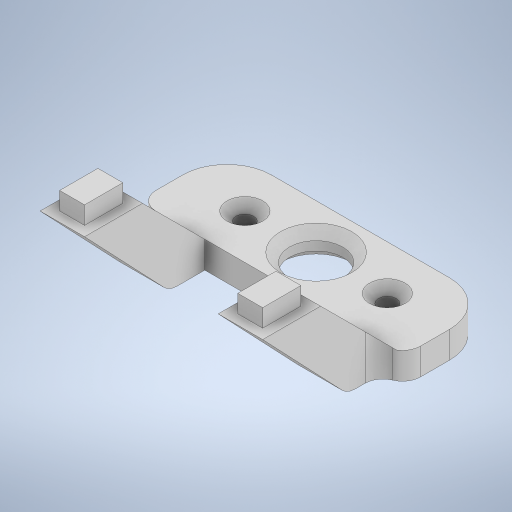
# Autodesk Inventor part: ServoUltrasonicMount
Saved by Autodesk Inventor 2024.2 (Build 282272000, 272)
## iProperties
Created: 2024-04-03
Part Number: ServoUltrasonicMount
Material: Generic
Document SubType Name: Modeling
Designer: ringl
Density: 1 g/cm^3
Appearance: Default
Author: ringl
Autodesk Inventor part; units mm, degrees
ref_plane "XZ Plane" through (0, 0, 0) normal (0, 1, 0) x (-1, 0, 0)
ref_plane "XY Plane" through (0, 0, 0) normal (0, 0, 1) x (1, 0, 0)
sketch "Sketch1" plane through (0, 0, 0) normal (0, 1, 0) x (-1, 0, 0)
  line L0 (0, 0) -> (30, 0)
  line L1 (30, 0) -> (30, -10)
  line L2 (30, -10) -> (0, -10)
  line L3 (0, -10) -> (0, 0)
  dimension "d0" = 30
  dimension "d1" = 10
  constraints: 8 end point, 2 parallel, 1 horizontal, 1 perpendicular
  measures "d0" distance of L1.end L2.end
  measures "d1" distance of L0.end L1.end
extrude "Extrusion1" add sketch "Sketch1" along normal blind 3
ref_plane "Work Plane2" through (-2.5, 0, 0) normal (1, 0, 0) x (0, 1, 0)
sketch "Sketch3" plane through (-2.5, 0, 0) normal (1, 0, 0) x (0, 1, 0)
  line L0 (3, -10) -> (3, 0) projected
  line L1 (3, 0) -> (10, 7)
  line L2 (10, 7) -> (10, 13.5)
  line L3 (10, 13.5) -> (0, 4)
  line L4 (0, 4) -> (0, 0)
  line L5 (0, 0) -> (3, 0) projected
  line L6 (3, 0) -> (0, 0)
  dimension "d13" = 4
  dimension "d14" = 6.5
  dimension "d15" = 45
  dimension "d16" = 10
  constraints: 10 end point, 2 parallel, 1 horizontal
  measures "d13" distance of L3.end L4.end
  measures "d14" distance of L1.end L2.end
  measures "d15" angle of L4 L1
  measures "d16" distance between parallel lines of L4 L2
extrude "Extrusion3" add sketch "Sketch3" against normal blind 5
ref_plane "Work Plane3" through (-15, 0, 0) normal (1, 0, 0) x (0, 1, 0)
fillet "Fillet2" radius 2 1 edges at (-5, 0, 4)
fillet "Fillet3" radius 2 4 edges at (-30, 1.5, 0) (-7.5, 1.5, 0) (-2.5, 1.5, 0) (0, 1.5, 0)
fillet "Fillet4" radius 5 2 edges at (-30, 1.5, -10) (0, 1.5, -10)
sketch "Sketch5" plane through (-2.5, 10, 13.5) normal (0, 1, 0) x (1, 0, 0)
  line L0 (-1.1, 5.4) -> (-3.9, 5.4)
  line L1 (-3.9, 5.4) -> (-3.9, 1.1)
  line L2 (-3.9, 1.1) -> (-1.1, 1.1)
  line L3 (-1.1, 1.1) -> (-1.1, 5.4)
  line L4 (-5, 0) -> (-5, 6.5) projected
  line L5 (0, 6.5) -> (-5, 6.5) projected
  point P0 (2.5, 13.5)
  dimension "d26" = 2.8
  dimension "d27" = 4.3
  dimension "d28" = 1.1
  dimension "d29" = 1.1
  constraints: 8 end point, 2 parallel, 1 horizontal, 1 perpendicular
  measures "d26" distance of L2.end L1.end
  measures "d27" distance of L1.end L0.end
  measures "d28" distance between parallel lines of L4 L1
  measures "d29" distance between parallel lines of L5 L0
extrude "Extrusion4" add sketch "Sketch5" along normal blind 2
mirror "Mirror2" about plane through (-15, 0, 0) normal (1, 0, 0) of "Extrusion3", "Extrusion4"
sketch "Sketch6" plane through (0, 3, 0) normal (0, 1, 0) x (1, 0, 0)
  circle A0 centre (-15, 5) radius 3
  line L0 (-5, 10) -> (-25, 10) projected
  line L1 (0, 1.7081) -> (0, 5) projected
  point P0 (0, 0)
  dimension "d32" = 6
  dimension "d33" = 5
  dimension "d34" = 15
  constraints: 1 centre point
  measures "d32" diameter of A0
  measures "d33" distance from line of L0 A0.centre
  measures "d34" distance from line of A0.centre L1
extrude "Extrusion5" cut sketch "Sketch6" against normal through all
chamfer "Chamfer1" distance 1 angle 45 1 edges at (-18, 3, -5)
sketch "Sketch7" plane through (0, 3, 0) normal (0, 1, 0) x (1, 0, 0)
  circle A0 centre (-23, 5) radius 1
  circle A1 centre (-7, 5) radius 1
  line L0 (-5, 10) -> (-25, 10) projected
  circle A2 centre (-15, 5) radius 3 projected
  point P0 (0, 0)
  dimension "d40" = 2
  dimension "d41" = 2
  dimension "d42" = 5
  dimension "d43" = 5
  dimension "d44" = 8
  dimension "d45" = 8
  constraints: 2 centre point
  measures "d40" diameter of A0
  measures "d41" diameter of A1
  measures "d42" distance from line of L0 A1.centre
  measures "d43" distance from line of L0 A0.centre
  measures "d44" distance of A2.centre A1.centre
  measures "d45" distance of A0.centre A2.centre
extrude "Extrusion6" cut sketch "Sketch7" against normal through all contours A0 | A1
chamfer "Chamfer2" distance 1 angle 45 2 edges at (-8, 3, -5) (-24, 3, -5)
fillet "Fillet5" radius 2 1 edges at (-25, 0, 4)
chamfer "Chamfer3" distance 1 angle 45 1 edges at (-18, 0, -5)
body "Solid1"
